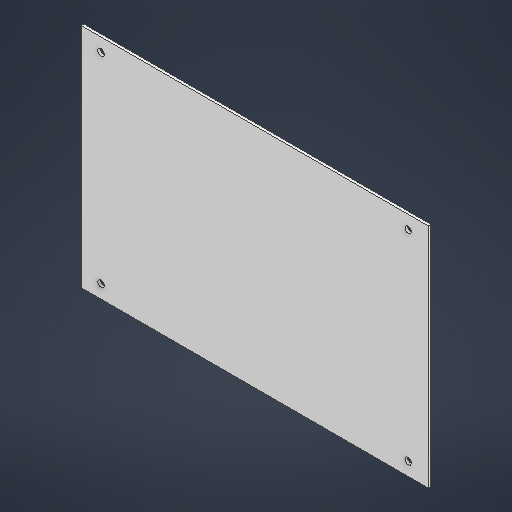
# Autodesk Inventor part: PlaqueBasPorte
Saved by Autodesk Inventor 2026.2 (Build 302298010, 298A)
## iProperties
Created: 2026-05-13
Part Number: PlaqueBasPorte
Material: Générique
Document SubType Name: Modeling
Designer: romai
Density: 1 g/cm^3
Appearance: Par défaut
Author: romai
Autodesk Inventor part; units mm, degrees
ref_plane "YZ Plane" through (0, 0, 0) normal (1, 0, 0) x (0, 1, 0)
ref_plane "XZ Plane" through (0, 0, 0) normal (0, 1, 0) x (-1, 0, 0)
ref_plane "XY Plane" through (0, 0, 0) normal (0, 0, 1) x (1, 0, 0)
sketch "Esquisse1" plane through (0, 0, 0) normal (0, 0, 1) x (1, 0, 0)
  line L0 (-130, -85) -> (130, -85)
  line L1 (130, -85) -> (130, 85)
  line L2 (130, 85) -> (-130, 85)
  line L3 (-130, 85) -> (-130, -85)
  line L4 (-130, -85) -> (130, 85) construction
  line L5 (130, -85) -> (-130, 85) construction
  line L6 (-117.5, -85) -> (117.5, -85)
  line L7 (117.5, -85) -> (117.5, 85)
  line L8 (117.5, 85) -> (-117.5, 85)
  line L9 (-117.5, 85) -> (-117.5, -85)
  line L10 (-117.5, -85) -> (117.5, 85) construction
  line L11 (117.5, -85) -> (-117.5, 85) construction
  circle A0 centre (-115, 75) radius 2.5
  circle A1 centre (-115, -75) radius 2.5
  circle A2 centre (115, -75) radius 2.5
  circle A3 centre (115, 75) radius 2.5
  point P0 (0, 0)
  dimension "d0" = 260
  dimension "d1" = 170
  dimension "d2" = 12.5
  dimension "d3" = 5
  dimension "d4" = 5
  dimension "d5" = 5
  dimension "d6" = 5
  dimension "d7" = 10
  dimension "d8" = 10
  dimension "d9" = 10
  dimension "d10" = 10
  constraints: 24 end point, 4 centre point, 4 midpoint, 4 parallel, 4 tangent, 2 horizontal, 2 perpendicular, 1 point on line
  measures "d0" distance of L2.end L1.end
  measures "d1" distance of L1.end L0.end
  measures "d2" distance between parallel lines of L1 L7
  measures "d3" diameter of A0
  measures "d4" diameter of A1
  measures "d5" diameter of A2
  measures "d6" diameter of A3
  measures "d7" distance from line of L8 A0.centre
  measures "d8" distance from line of L8 A3.centre
  measures "d9" distance from line of L6 A1.centre
  measures "d10" distance from line of L6 A2.centre
extrude "Extrusion1" add sketch "Esquisse1" along normal blind 2
